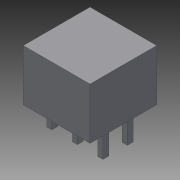
# Autodesk Inventor part: pin
Saved by Autodesk Inventor 2015 (Build 190159000, 159)
## iProperties
Created: 2015-10-12
Part Number: pin
Material: 一般
Document SubType Name: シート メタル
Designer: kenta
Density: 1 g/cm^3
Sheet Metal Rule: Default_mm
Appearance: 既定
Author: kenta
Autodesk Inventor part; units mm, degrees
ref_plane "YZ Plane" through (0, 0, 0) normal (1, 0, 0) x (0, 1, 0)
ref_plane "XZ Plane" through (0, 0, 0) normal (0, 1, 0) x (-1, 0, 0)
ref_plane "XY Plane" through (0, 0, 0) normal (0, 0, 1) x (1, 0, 0)
sketch "スケッチ1" plane through (0, 0, 0) normal (0, 0, 1) x (1, 0, 0)
  line L0 (-28.5941, 8.0239) -> (-27.6141, 8.0239)
  line L1 (-27.6141, 8.0239) -> (-27.6141, 6.8739)
  line L2 (-27.6141, 6.8739) -> (-28.5941, 6.8739)
  line L3 (-28.5941, 6.8739) -> (-28.5941, 8.0239)
  line L4 (-23.6141, 8.0239) -> (-22.6341, 8.0239)
  line L5 (-22.6341, 8.0239) -> (-22.6341, 6.8739)
  line L6 (-22.6341, 6.8739) -> (-23.6141, 6.8739)
  line L7 (-23.6141, 6.8739) -> (-23.6141, 8.0239)
  line L8 (-18.6341, 8.0239) -> (-17.6541, 8.0239)
  line L9 (-17.6541, 8.0239) -> (-17.6541, 6.8739)
  line L10 (-17.6541, 6.8739) -> (-18.6341, 6.8739)
  line L11 (-18.6341, 6.8739) -> (-18.6341, 8.0239)
  line L12 (-28.5941, 3.2739) -> (-27.6141, 3.2739)
  line L13 (-27.6141, 3.2739) -> (-27.6141, 2.1239)
  line L14 (-27.6141, 2.1239) -> (-28.5941, 2.1239)
  line L15 (-28.5941, 2.1239) -> (-28.5941, 3.2739)
  line L16 (-23.6141, 3.2739) -> (-22.6341, 3.2739)
  line L17 (-22.6341, 3.2739) -> (-22.6341, 2.1239)
  line L18 (-22.6341, 2.1239) -> (-23.6141, 2.1239)
  line L19 (-23.6141, 2.1239) -> (-23.6141, 3.2739)
  line L20 (-18.6341, 3.2739) -> (-17.6541, 3.2739)
  line L21 (-17.6541, 3.2739) -> (-17.6541, 2.1239)
  line L22 (-17.6541, 2.1239) -> (-18.6341, 2.1239)
  line L23 (-18.6341, 2.1239) -> (-18.6341, 3.2739)
  dimension "d2" = 0.98
  dimension "d3" = 1.15
  dimension "d4" = 0.98
  dimension "d5" = 1.15
  dimension "d6" = 0.98
  dimension "d7" = 1.15
  dimension "d8" = 0.98
  dimension "d9" = 1.15
  dimension "d10" = 0.98
  dimension "d11" = 1.15
  dimension "d12" = 0.98
  dimension "d13" = 1.15
  dimension "d14" = 4
  dimension "d15" = 0
  dimension "d16" = 0
  dimension "d17" = 4
  dimension "d18" = 0
  dimension "d19" = 0
  dimension "d20" = 3.6
  dimension "d21" = 4
  dimension "d22" = 0
  dimension "d23" = 0
  constraints: 48 end point, 12 parallel, 6 horizontal, 6 perpendicular
  measures "d2" distance of L0.start L0.end
  measures "d3" distance of L0.end L1.end
  measures "d4" distance of L4.start L4.end
  measures "d5" distance of L4.end L5.end
  measures "d6" distance of L8.start L8.end
  measures "d7" distance of L8.end L9.end
  measures "d8" distance of L15.end L13.start
  measures "d9" distance of L13.start L13.end
  measures "d10" distance of L16.start L17.start
  measures "d11" distance of L17.start L17.end
  measures "d12" distance of L20.start L21.start
  measures "d13" distance of L21.start L21.end
  measures "d14" distance between parallel lines of L7 L1
  measures "d15" distance between parallel lines of L0 L4
  measures "d16" distance between parallel lines of L4 L8
  measures "d17" distance between parallel lines of L5 L11
  measures "d18" distance between parallel lines of L3 L15
  measures "d19" distance between parallel lines of L21 L9
  measures "d20" distance between parallel lines of L12 L2
  measures "d21" distance between parallel lines of L13 L19
  measures "d22" distance between parallel lines of L14 L18
  measures "d23" distance between parallel lines of L18 L22
extrude "押し出し1" add sketch "スケッチ1" along normal blind 5
sketch "スケッチ2" plane through (0, 0, 5) normal (0, 0, 1) x (1, 0, 0)
  line L0 (-29.6241, 11.5739) -> (-16.6241, 11.5739)
  line L1 (-16.6241, 11.5739) -> (-16.6241, -1.4261)
  line L2 (-16.6241, -1.4261) -> (-29.6241, -1.4261)
  line L3 (-29.6241, -1.4261) -> (-29.6241, 11.5739)
  line L4 (-17.6541, 8.0239) -> (-18.6341, 8.0239) projected
  line L5 (-17.6541, 2.1239) -> (-17.6541, 3.2739) projected
  line L6 (-28.5941, 3.2739) -> (-28.5941, 2.1239) projected
  point P0 (0, 0)
  dimension "d26" = 13
  dimension "d27" = 13
  dimension "d28" = 3.55
  dimension "d29" = 10.94
  dimension "d30" = 1.03
  constraints: 8 end point, 2 parallel, 1 horizontal, 1 perpendicular
  measures "d26" distance of L0.start L0.end
  measures "d27" distance of L0.end L1.end
  measures "d28" distance between parallel lines of L4 L0
  measures "d29" distance between parallel lines of L5 L6
  measures "d30" distance between parallel lines of L6 L3
extrude "押し出し2" add sketch "スケッチ2" along normal blind 10
equation "\"BendRadius\" = Thickness"
equation "\"BendReliefWidth\" = Thickness"
equation "\"BendReliefDepth\" = 0.5 * Thickness"
equation "\"CornerReliefSize\" = 4 * Thickness"
equation "\"MinimumRemnant\" = 2 * Thickness"
equation "\"TransitionRadius\" = BendRadius"
equation "\"JacobiRadiusSize\" = BendRadius"
equation "\"GapSize\" = Thickness"
equation "\"Thickness\" = 0.5"
